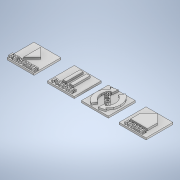
# Autodesk Inventor part: buttons
Saved by Autodesk Inventor 2022.1 (Build 261234020, 234B)
## iProperties
Created: 2021-11-01
Part Number: buttons
Material: Generico
Document SubType Name: Modeling
Designer: chicco
Density: 1 g/cm^3
Appearance: Default
Author: chicco
Autodesk Inventor part; units mm, degrees
ref_plane "YZ Plane" through (0, 0, 0) normal (1, 0, 0) x (0, 1, 0)
ref_plane "XZ Plane" through (0, 0, 0) normal (0, 1, 0) x (-1, 0, 0)
ref_plane "XY Plane" through (0, 0, 0) normal (0, 0, 1) x (1, 0, 0)
sketch "Schizzo1" plane through (0, 0, 0) normal (0, 1, 0) x (-1, 0, 0)
  line L0 (4.6852, 27.8019) -> (-9.8148, 27.8019)
  line L1 (-9.8148, 27.8019) -> (-9.8148, 13.3019)
  line L2 (-9.8148, 13.3019) -> (4.6852, 13.3019)
  line L3 (4.6852, 13.3019) -> (4.6852, 27.8019)
  line L4 (-17.0713, 27.8038) -> (-31.5713, 27.8038)
  line L5 (-31.5713, 27.8038) -> (-31.5713, 13.3038)
  line L6 (-31.5713, 13.3038) -> (-17.0713, 13.3038)
  line L7 (-17.0713, 13.3038) -> (-17.0713, 27.8038)
  line L8 (-55.7694, 27.7904) -> (-70.2694, 27.7904)
  line L9 (-70.2694, 27.7904) -> (-70.2694, 13.2904)
  line L10 (-70.2694, 13.2904) -> (-55.7694, 13.2904)
  line L11 (-55.7694, 13.2904) -> (-55.7694, 27.7904)
  line L12 (4.6852, 13.3019) -> (-76.0307, 13.3019) construction
  line L13 (-35.4166, 27.7793) -> (-49.9166, 27.7793)
  line L14 (-49.9166, 27.7793) -> (-49.9166, 13.2793)
  line L15 (-49.9166, 13.2793) -> (-35.4166, 13.2793)
  line L16 (-35.4166, 13.2793) -> (-35.4166, 27.7793)
  point P0 (0, 0)
  dimension "d0" = 14.5
  dimension "d1" = 14.5
  dimension "d6" = 14.5
  dimension "d7" = 14.5
  dimension "d8" = 14.5
  dimension "d9" = 14.5
  dimension "d10" = 14.5
  dimension "d11" = 14.5
  constraints: 34 end point, 8 parallel, 5 horizontal, 4 perpendicular
  measures "d0" distance of L2.end L1.end
  measures "d1" distance of L0.start L2.end
  measures "d6" distance of L6.end L5.end
  measures "d7" distance of L4.start L6.end
  measures "d8" distance of L10.end L9.end
  measures "d9" distance of L8.start L10.end
  measures "d10" distance of L16.start L14.end
  measures "d11" distance of L16.end L16.start
extrude "Estrusione1" add sketch "Schizzo1" along normal blind 1
sketch "Schizzo2" plane through (0, 1, 0) normal (0, 1, 0) x (1, 0, 0)
  line L0 (0.9348, -18.5902) -> (3.7499, -18.5902) construction
  line L1 (3.7499, -18.5902) -> (3.7499, -20.3496) construction
  line L2 (3.7499, -20.3496) -> (0.9348, -20.3496) construction
  line L3 (0.9348, -20.3496) -> (0.9348, -18.5902) construction
  line L4 (-7.5474, -24.5477) -> (12.5843, -24.5477) construction
  line L5 (12.5843, -24.5477) -> (12.5843, -27.7034) construction
  line L6 (12.5843, -27.7034) -> (-7.5474, -27.7034) construction
  line L7 (-7.5474, -27.7034) -> (-7.5474, -24.5477) construction
  line L8 (14.2097, -28.0868) -> (34.3415, -28.0868) construction
  line L9 (34.3415, -28.0868) -> (34.3415, -24.1124) construction
  line L10 (34.3415, -24.1124) -> (14.2097, -24.1124) construction
  line L11 (14.2097, -24.1124) -> (14.2097, -28.0868) construction
  line L12 (-3.7448, -25.0033) -> (81.6896, -25.0033) construction
  line L13 (23.1791, -18.5734) -> (25.9942, -18.5734) construction
  line L14 (25.9942, -18.5734) -> (25.9942, -20.3328) construction
  line L15 (25.9942, -20.3328) -> (23.1791, -20.3328) construction
  line L16 (23.1791, -20.3328) -> (23.1791, -18.5734) construction
  line L17 (41.3289, -21.4494) -> (41.3289, -19.69) construction
  line L18 (41.3289, -19.69) -> (44.2154, -19.69) construction
  line L19 (44.2154, -19.69) -> (44.2154, -21.4494) construction
  line L20 (44.2154, -21.4494) -> (41.3289, -21.4494) construction
  line L21 (36.8214, -12.3845) -> (34.0111, -15.1947) construction
  line L22 (34.0111, -15.1947) -> (48.2464, -29.4301) construction
  line L23 (48.2464, -29.4301) -> (51.0567, -26.6198) construction
  line L24 (51.0567, -26.6198) -> (36.8214, -12.3845) construction
  line L25 (52.8656, -24.1572) -> (52.8656, -28.1316) construction
  line L26 (52.8656, -28.1316) -> (72.9973, -28.1316) construction
  line L27 (72.9973, -28.1316) -> (72.9973, -24.1572) construction
  line L28 (72.9973, -24.1572) -> (52.8656, -24.1572) construction
  line L29 (61.9799, -18.2818) -> (61.9799, -15.4667) construction
  line L30 (61.9799, -15.4667) -> (63.7393, -15.4667) construction
  line L31 (63.7393, -15.4667) -> (63.7393, -18.2818) construction
  line L32 (63.7393, -18.2818) -> (61.9799, -18.2818) construction
  line L33 (58.2477, -18.6857) -> (58.2477, -24.1572)
  line L34 (67.3768, -24.1572) -> (67.3768, -18.6857)
  line L35 (67.3768, -18.6857) -> (58.2477, -18.6857)
  line L36 (58.2477, -24.1572) -> (67.3768, -24.1572)
  line L37 (5.1082, -19.4699) -> (0.4984, -24.0798)
  line L38 (0.4984, -24.0798) -> (0.4984, -14.8601)
  line L39 (0.4984, -14.8601) -> (5.1082, -19.4699)
  line L40 (-4.5072, -27.2255) -> (-4.5072, -25.0255)
  line L41 (-4.5072, -25.0255) -> (-3.3743, -25.0255)
  spline S0 degree 2 poles (-3.3743, -25.0255) (-3.061, -25.0255) (-2.7264, -25.1335) (-2.5231, -25.4257) (-2.5231, -25.6353) knots 0 0 0 1 2 3 3 3
  spline S1 degree 2 poles (-2.5231, -25.6353) (-2.5231, -25.8195) (-2.6798, -26.0842) (-2.8153, -26.1668) knots 0 0 0 1 2 2 2
  spline S2 degree 2 poles (-2.8153, -26.1668) (-2.9022, -26.2197) (-3.0546, -26.2536) knots 0 0 0 1 1 1
  spline S3 degree 2 poles (-3.0546, -26.2536) (-2.9339, -26.2938) (-2.8767, -26.3341) knots 0 0 0 1 1 1
  spline S4 degree 2 poles (-2.8767, -26.3341) (-2.8407, -26.3616) (-2.6989, -26.5395) (-2.6735, -26.5882) knots 0 0 0 1 2 2 2
  line L42 (-2.6735, -26.5882) -> (-2.3453, -27.2255)
  line L43 (-2.3453, -27.2255) -> (-3.1139, -27.2255)
  line L44 (-3.1139, -27.2255) -> (-3.476, -26.5522)
  spline S5 degree 2 poles (-3.476, -26.5522) (-3.5437, -26.423) (-3.5967, -26.3828) knots 0 0 0 1 1 1
  spline S6 degree 2 poles (-3.5967, -26.3828) (-3.6708, -26.332) (-3.7639, -26.332) knots 0 0 0 1 1 1
  line L45 (-3.7639, -26.332) -> (-3.8232, -26.332)
  line L46 (-3.8232, -26.332) -> (-3.8232, -27.2255)
  line L47 (-3.8232, -27.2255) -> (-4.5072, -27.2255)
  line L48 (-3.8232, -25.9169) -> (-3.5374, -25.9169)
  spline S7 degree 2 poles (-3.5374, -25.9169) (-3.4929, -25.9169) (-3.3595, -25.8873) knots 0 0 0 1 1 1
  spline S8 degree 2 poles (-3.3595, -25.8873) (-3.2918, -25.8725) (-3.2071, -25.7624) (-3.2071, -25.6904) knots 0 0 0 1 2 2 2
  spline S9 degree 2 poles (-3.2071, -25.6904) (-3.2071, -25.5845) (-3.3405, -25.4702) (-3.5268, -25.4702) knots 0 0 0 1 2 2 2
  line L49 (-3.5268, -25.4702) -> (-3.8232, -25.4702)
  line L50 (-3.8232, -25.4702) -> (-3.8232, -25.9169)
  line L51 (-2.1251, -25.0255) -> (-0.3041, -25.0255)
  line L52 (-0.3041, -25.0255) -> (-0.3041, -25.4956)
  line L53 (-0.3041, -25.4956) -> (-1.4432, -25.4956)
  line L54 (-1.4432, -25.4956) -> (-1.4432, -25.845)
  line L55 (-1.4432, -25.845) -> (-0.3867, -25.845)
  line L56 (-0.3867, -25.845) -> (-0.3867, -26.2938)
  line L57 (-0.3867, -26.2938) -> (-1.4432, -26.2938)
  line L58 (-1.4432, -26.2938) -> (-1.4432, -26.7279)
  line L59 (-1.4432, -26.7279) -> (-0.2702, -26.7279)
  line L60 (-0.2702, -26.7279) -> (-0.2702, -27.2255)
  line L61 (-0.2702, -27.2255) -> (-2.1251, -27.2255)
  line L62 (-2.1251, -27.2255) -> (-2.1251, -25.0255)
  line L63 (-0.0225, -26.4971) -> (0.6255, -26.4569)
  spline S10 degree 2 poles (0.6255, -26.4569) (0.6466, -26.6157) (0.7102, -26.6983) knots 0 0 0 1 1 1
  spline S11 degree 2 poles (0.7102, -26.6983) (0.816, -26.8317) (1.013, -26.8317) knots 0 0 0 1 1 1
  spline S12 degree 2 poles (1.013, -26.8317) (1.1569, -26.8317) (1.3158, -26.694) (1.3158, -26.6051) knots 0 0 0 1 2 2 2
  spline S13 degree 2 poles (1.3158, -26.6051) (1.3158, -26.5204) (1.2395, -26.4527) knots 0 0 0 1 1 1
  spline S14 degree 2 poles (1.2395, -26.4527) (1.1654, -26.3849) (0.8923, -26.3235) knots 0 0 0 1 1 1
  spline S15 degree 2 poles (0.8923, -26.3235) (0.4434, -26.224) (0.2528, -26.0567) knots 0 0 0 1 1 1
  spline S16 degree 2 poles (0.2528, -26.0567) (0.0601, -25.8894) (0.0601, -25.6311) knots 0 0 0 1 1 1
  spline S17 degree 2 poles (0.0601, -25.6311) (0.0601, -25.4617) (0.257, -25.161) (0.653, -24.9874) (0.996, -24.9874) knots 0 0 0 1 2 3 3 3
  spline S18 degree 2 poles (0.996, -24.9874) (1.4195, -24.9874) (1.862, -25.3008) (1.9044, -25.6438) knots 0 0 0 1 2 2 2
  line L64 (1.9044, -25.6438) -> (1.2628, -25.6819)
  spline S19 degree 2 poles (1.2628, -25.6819) (1.2374, -25.5337) (1.0722, -25.3982) (0.9283, -25.3982) knots 0 0 0 1 2 2 2
  spline S20 degree 2 poles (0.9283, -25.3982) (0.8097, -25.3982) (0.689, -25.4977) (0.689, -25.5718) knots 0 0 0 1 2 2 2
  spline S21 degree 2 poles (0.689, -25.5718) (0.689, -25.6226) (0.7398, -25.665) knots 0 0 0 1 1 1
  spline S22 degree 2 poles (0.7398, -25.665) (0.7885, -25.7094) (0.9685, -25.7454) knots 0 0 0 1 1 1
  spline S23 degree 2 poles (0.9685, -25.7454) (1.4153, -25.8428) (1.8006, -26.0398) (1.9764, -26.3298) (1.9764, -26.5098) knots 0 0 0 1 2 3 3 3
  spline S24 degree 2 poles (1.9764, -26.5098) (1.9764, -26.7216) (1.7414, -27.0794) (1.3221, -27.2636) (1.0003, -27.2636) knots 0 0 0 1 2 3 3 3
  spline S25 degree 2 poles (1.0003, -27.2636) (0.4391, -27.2636) (0.0051, -26.8317) (-0.0225, -26.4971) knots 0 0 0 1 2 2 2
  line L65 (3.7529, -25.0255) -> (4.4305, -25.0255)
  line L66 (4.4305, -25.0255) -> (4.4305, -26.3362)
  spline S26 degree 2 poles (4.4305, -26.3362) (4.4305, -26.531) (4.3098, -26.8783) (4.0493, -27.1366) (3.9054, -27.1895) knots 0 0 0 1 2 3 3 3
  spline S27 degree 2 poles (3.9054, -27.1895) (3.7084, -27.2636) (3.4289, -27.2636) knots 0 0 0 1 1 1
  spline S28 degree 2 poles (3.4289, -27.2636) (3.268, -27.2636) (2.889, -27.2192) (2.6328, -27.0858) (2.421, -26.8401) (2.3829, -26.7089) knots 0 0 0 1 2 3 4 4 4
  spline S29 degree 2 poles (2.3829, -26.7089) (2.3194, -26.4992) (2.3194, -26.3362) knots 0 0 0 1 1 1
  line L67 (2.3194, -26.3362) -> (2.3194, -25.0255)
  line L68 (2.3194, -25.0255) -> (2.997, -25.0255)
  line L69 (2.997, -25.0255) -> (2.997, -26.368)
  spline S30 degree 2 poles (2.997, -26.368) (2.997, -26.5479) (3.1981, -26.7512) (3.376, -26.7512) knots 0 0 0 1 2 2 2
  spline S31 degree 2 poles (3.376, -26.7512) (3.5517, -26.7512) (3.7529, -26.5522) (3.7529, -26.368) knots 0 0 0 1 2 2 2
  line L70 (3.7529, -26.368) -> (3.7529, -25.0255)
  line L71 (4.873, -25.0255) -> (5.7687, -25.0255)
  line L72 (5.7687, -25.0255) -> (6.1117, -26.3637)
  line L73 (6.1117, -26.3637) -> (6.4526, -25.0255)
  line L74 (6.4526, -25.0255) -> (7.3462, -25.0255)
  line L75 (7.3462, -25.0255) -> (7.3462, -27.2255)
  line L76 (7.3462, -27.2255) -> (6.7893, -27.2255)
  line L77 (6.7893, -27.2255) -> (6.7893, -25.5464)
  line L78 (6.7893, -25.5464) -> (6.3616, -27.2255)
  line L79 (6.3616, -27.2255) -> (5.8576, -27.2255)
  line L80 (5.8576, -27.2255) -> (5.4299, -25.5464)
  line L81 (5.4299, -25.5464) -> (5.4299, -27.2255)
  line L82 (5.4299, -27.2255) -> (4.873, -27.2255)
  line L83 (4.873, -27.2255) -> (4.873, -25.0255)
  line L84 (7.7824, -25.0255) -> (9.6033, -25.0255)
  line L85 (9.6033, -25.0255) -> (9.6033, -25.4956)
  line L86 (9.6033, -25.4956) -> (8.4642, -25.4956)
  line L87 (8.4642, -25.4956) -> (8.4642, -25.845)
  line L88 (8.4642, -25.845) -> (9.5208, -25.845)
  line L89 (9.5208, -25.845) -> (9.5208, -26.2938)
  line L90 (9.5208, -26.2938) -> (8.4642, -26.2938)
  line L91 (8.4642, -26.2938) -> (8.4642, -26.7279)
  line L92 (8.4642, -26.7279) -> (9.6372, -26.7279)
  line L93 (9.6372, -26.7279) -> (9.6372, -27.2255)
  line L94 (9.6372, -27.2255) -> (7.7824, -27.2255)
  line L95 (7.7824, -27.2255) -> (7.7824, -25.0255)
  line L96 (23.4846, -24.063) -> (21.6406, -24.063)
  line L97 (21.6406, -24.063) -> (21.6406, -14.8433)
  line L98 (21.6406, -14.8433) -> (23.4846, -14.8433)
  line L99 (23.4846, -14.8433) -> (23.4846, -24.063)
  line L100 (27.1724, -24.063) -> (25.3285, -24.063)
  line L101 (25.3285, -24.063) -> (25.3285, -14.8433)
  line L102 (25.3285, -14.8433) -> (27.1724, -14.8433)
  line L103 (27.1724, -14.8433) -> (27.1724, -24.063)
  line L104 (18.6888, -24.9996) -> (19.8195, -24.9996)
  spline S32 degree 2 poles (19.8195, -24.9996) (20.1879, -24.9996) (20.5563, -25.3511) (20.5563, -25.675) knots 0 0 0 1 2 2 2
  spline S33 degree 2 poles (20.5563, -25.675) (20.5563, -26.0096) (20.1561, -26.3844) (19.7454, -26.3844) knots 0 0 0 1 2 2 2
  line L105 (19.7454, -26.3844) -> (19.3727, -26.3844)
  line L106 (19.3727, -26.3844) -> (19.3727, -27.1996)
  line L107 (19.3727, -27.1996) -> (18.6888, -27.1996)
  line L108 (18.6888, -27.1996) -> (18.6888, -24.9996)
  line L109 (19.3727, -25.9376) -> (19.5379, -25.9376)
  spline S34 degree 2 poles (19.5379, -25.9376) (19.7348, -25.9376) (19.8936, -25.8) (19.8936, -25.6941) knots 0 0 0 1 2 2 2
  spline S35 degree 2 poles (19.8936, -25.6941) (19.8936, -25.5903) (19.7559, -25.4464) (19.5654, -25.4464) knots 0 0 0 1 2 2 2
  line L110 (19.5654, -25.4464) -> (19.3727, -25.4464)
  line L111 (19.3727, -25.4464) -> (19.3727, -25.9376)
  line L112 (22.2651, -26.8354) -> (21.4922, -26.8354)
  line L113 (21.4922, -26.8354) -> (21.3842, -27.1996)
  line L114 (21.3842, -27.1996) -> (20.6897, -27.1996)
  line L115 (20.6897, -27.1996) -> (21.5176, -24.9996)
  line L116 (21.5176, -24.9996) -> (22.2609, -24.9996)
  line L117 (22.2609, -24.9996) -> (23.0867, -27.1996)
  line L118 (23.0867, -27.1996) -> (22.3752, -27.1996)
  line L119 (22.3752, -27.1996) -> (22.2651, -26.8354)
  line L120 (22.1232, -26.359) -> (21.8818, -25.5692)
  line L121 (21.8818, -25.5692) -> (21.6405, -26.359)
  line L122 (21.6405, -26.359) -> (22.1232, -26.359)
  line L123 (24.7404, -24.9996) -> (25.4179, -24.9996)
  line L124 (25.4179, -24.9996) -> (25.4179, -26.3103)
  spline S36 degree 2 poles (25.4179, -26.3103) (25.4179, -26.5051) (25.2972, -26.8523) (25.0368, -27.1107) (24.8928, -27.1636) knots 0 0 0 1 2 3 3 3
  spline S37 degree 2 poles (24.8928, -27.1636) (24.6959, -27.2377) (24.4164, -27.2377) knots 0 0 0 1 1 1
  spline S38 degree 2 poles (24.4164, -27.2377) (24.2555, -27.2377) (23.8764, -27.1932) (23.6202, -27.0598) (23.4085, -26.8142) (23.3704, -26.6829) knots 0 0 0 1 2 3 4 4 4
  spline S39 degree 2 poles (23.3704, -26.6829) (23.3069, -26.4733) (23.3069, -26.3103) knots 0 0 0 1 1 1
  line L125 (23.3069, -26.3103) -> (23.3069, -24.9996)
  line L126 (23.3069, -24.9996) -> (23.9844, -24.9996)
  line L127 (23.9844, -24.9996) -> (23.9844, -26.342)
  spline S40 degree 2 poles (23.9844, -26.342) (23.9844, -26.522) (24.1856, -26.7253) (24.3635, -26.7253) knots 0 0 0 1 2 2 2
  spline S41 degree 2 poles (24.3635, -26.7253) (24.5392, -26.7253) (24.7404, -26.5262) (24.7404, -26.342) knots 0 0 0 1 2 2 2
  line L128 (24.7404, -26.342) -> (24.7404, -24.9996)
  line L129 (25.7482, -26.4712) -> (26.3962, -26.431)
  spline S42 degree 2 poles (26.3962, -26.431) (26.4174, -26.5898) (26.4809, -26.6724) knots 0 0 0 1 1 1
  spline S43 degree 2 poles (26.4809, -26.6724) (26.5867, -26.8057) (26.7837, -26.8057) knots 0 0 0 1 1 1
  spline S44 degree 2 poles (26.7837, -26.8057) (26.9277, -26.8057) (27.0865, -26.6681) (27.0865, -26.5792) knots 0 0 0 1 2 2 2
  spline S45 degree 2 poles (27.0865, -26.5792) (27.0865, -26.4945) (27.0102, -26.4267) knots 0 0 0 1 1 1
  spline S46 degree 2 poles (27.0102, -26.4267) (26.9361, -26.359) (26.663, -26.2976) knots 0 0 0 1 1 1
  spline S47 degree 2 poles (26.663, -26.2976) (26.2141, -26.198) (26.0235, -26.0308) knots 0 0 0 1 1 1
  spline S48 degree 2 poles (26.0235, -26.0308) (25.8308, -25.8635) (25.8308, -25.6052) knots 0 0 0 1 1 1
  spline S49 degree 2 poles (25.8308, -25.6052) (25.8308, -25.4358) (26.0277, -25.1351) (26.4237, -24.9615) (26.7667, -24.9615) knots 0 0 0 1 2 3 3 3
  spline S50 degree 2 poles (26.7667, -24.9615) (27.1902, -24.9615) (27.6328, -25.2749) (27.6751, -25.6179) knots 0 0 0 1 2 2 2
  line L130 (27.6751, -25.6179) -> (27.0335, -25.656)
  spline S51 degree 2 poles (27.0335, -25.656) (27.0081, -25.5078) (26.843, -25.3723) (26.699, -25.3723) knots 0 0 0 1 2 2 2
  spline S52 degree 2 poles (26.699, -25.3723) (26.5804, -25.3723) (26.4597, -25.4718) (26.4597, -25.5459) knots 0 0 0 1 2 2 2
  spline S53 degree 2 poles (26.4597, -25.5459) (26.4597, -25.5967) (26.5105, -25.6391) knots 0 0 0 1 1 1
  spline S54 degree 2 poles (26.5105, -25.6391) (26.5592, -25.6835) (26.7392, -25.7195) knots 0 0 0 1 1 1
  spline S55 degree 2 poles (26.7392, -25.7195) (27.186, -25.8169) (27.5713, -26.0138) (27.7471, -26.3039) (27.7471, -26.4839) knots 0 0 0 1 2 3 3 3
  spline S56 degree 2 poles (27.7471, -26.4839) (27.7471, -26.6956) (27.5121, -27.0535) (27.0928, -27.2377) (26.771, -27.2377) knots 0 0 0 1 2 3 3 3
  spline S57 degree 2 poles (26.771, -27.2377) (26.2098, -27.2377) (25.7758, -26.8057) (25.7482, -26.4712) knots 0 0 0 1 2 2 2
  line L131 (28.088, -24.9996) -> (29.909, -24.9996)
  line L132 (29.909, -24.9996) -> (29.909, -25.4697)
  line L133 (29.909, -25.4697) -> (28.7698, -25.4697)
  line L134 (28.7698, -25.4697) -> (28.7698, -25.819)
  line L135 (28.7698, -25.819) -> (29.8264, -25.819)
  line L136 (29.8264, -25.819) -> (29.8264, -26.2679)
  line L137 (29.8264, -26.2679) -> (28.7698, -26.2679)
  line L138 (28.7698, -26.2679) -> (28.7698, -26.702)
  line L139 (28.7698, -26.702) -> (29.9429, -26.702)
  line L140 (29.9429, -26.702) -> (29.9429, -27.1996)
  line L141 (29.9429, -27.1996) -> (28.088, -27.1996)
  line L142 (28.088, -27.1996) -> (28.088, -24.9996)
  spline S58 degree 2 poles (48.936, -20.2517) (48.936, -21.8269) (48.2903, -23.226) knots 0 0 0 1 1 1
  spline S59 degree 2 poles (48.2903, -23.226) (47.6054, -24.6838) (46.3726, -25.584) knots 0 0 0 1 1 1
  line L143 (46.3726, -25.584) -> (47.4586, -26.4352)
  line L144 (47.4586, -26.4352) -> (43.9658, -27.3744)
  line L145 (43.9658, -27.3744) -> (44.2886, -23.9011)
  line L146 (44.2886, -23.9011) -> (45.267, -24.6741)
  spline S60 degree 2 poles (45.267, -24.6741) (46.7835, -23.3337) (46.7835, -20.9464) knots 0 0 0 1 1 1
  spline S61 degree 2 poles (46.7835, -20.9464) (46.7835, -17.884) (43.8679, -16.1621) knots 0 0 0 1 1 1
  line L147 (43.8679, -16.1621) -> (45.1007, -13.765)
  spline S62 degree 2 poles (45.1007, -13.765) (46.9009, -14.6358) (47.938, -16.4556) knots 0 0 0 1 1 1
  spline S63 degree 2 poles (47.938, -16.4556) (48.936, -18.1971) (48.936, -20.2517) knots 0 0 0 1 1 1
  line L148 (41.4611, -24.9774) -> (40.2283, -27.3744)
  spline S64 degree 2 poles (40.2283, -27.3744) (38.4379, -26.5037) (37.4008, -24.6838) knots 0 0 0 1 1 1
  spline S65 degree 2 poles (37.4008, -24.6838) (36.393, -22.9423) (36.393, -20.8877) knots 0 0 0 1 1 1
  spline S66 degree 2 poles (36.393, -20.8877) (36.393, -19.3125) (37.0485, -17.9134) knots 0 0 0 1 1 1
  spline S67 degree 2 poles (37.0485, -17.9134) (37.7334, -16.4556) (38.9564, -15.5555) knots 0 0 0 1 1 1
  line L149 (38.9564, -15.5555) -> (37.8704, -14.6945)
  line L150 (37.8704, -14.6945) -> (41.3633, -13.765)
  line L151 (41.3633, -13.765) -> (41.0404, -17.2383)
  line L152 (41.0404, -17.2383) -> (40.062, -16.4654)
  spline S68 degree 2 poles (40.062, -16.4654) (38.5455, -17.8058) (38.5455, -20.193) knots 0 0 0 1 1 1
  spline S69 degree 2 poles (38.5455, -20.193) (38.5455, -23.2554) (41.4611, -24.9774) knots 0 0 0 1 1 1
  line L153 (39.0842, -17.9831) -> (39.5708, -18.4128)
  spline S70 degree 2 poles (39.5708, -18.4128) (39.4735, -18.5401) (39.46, -18.6434) knots 0 0 0 1 1 1
  spline S71 degree 2 poles (39.46, -18.6434) (39.4406, -18.8126) (39.5798, -18.9519) knots 0 0 0 1 1 1
  spline S72 degree 2 poles (39.5798, -18.9519) (39.6816, -19.0537) (39.8912, -19.0686) (39.9541, -19.0058) knots 0 0 0 1 2 2 2
  spline S73 degree 2 poles (39.9541, -19.0058) (40.014, -18.9459) (40.008, -18.8441) knots 0 0 0 1 1 1
  spline S74 degree 2 poles (40.008, -18.8441) (40.0035, -18.7437) (39.8538, -18.5072) knots 0 0 0 1 1 1
  spline S75 degree 2 poles (39.8538, -18.5072) (39.6068, -18.1194) (39.5903, -17.8664) knots 0 0 0 1 1 1
  spline S76 degree 2 poles (39.5903, -17.8664) (39.5723, -17.6118) (39.755, -17.4292) knots 0 0 0 1 1 1
  spline S77 degree 2 poles (39.755, -17.4292) (39.8748, -17.3094) (40.2266, -17.236) (40.6294, -17.3932) (40.8719, -17.6358) knots 0 0 0 1 2 3 3 3
  spline S78 degree 2 poles (40.8719, -17.6358) (41.1714, -17.9352) (41.2627, -18.4697) (41.0501, -18.7422) knots 0 0 0 1 2 2 2
  line L154 (41.0501, -18.7422) -> (40.5695, -18.3155)
  spline S79 degree 2 poles (40.5695, -18.3155) (40.6563, -18.1928) (40.6354, -17.9801) (40.5336, -17.8783) knots 0 0 0 1 2 2 2
  spline S80 degree 2 poles (40.5336, -17.8783) (40.4497, -17.7945) (40.294, -17.7795) (40.2416, -17.8319) knots 0 0 0 1 2 2 2
  spline S81 degree 2 poles (40.2416, -17.8319) (40.2057, -17.8678) (40.2117, -17.9337) knots 0 0 0 1 1 1
  spline S82 degree 2 poles (40.2117, -17.9337) (40.2146, -17.9996) (40.3165, -18.1523) knots 0 0 0 1 1 1
  spline S83 degree 2 poles (40.3165, -18.1523) (40.5635, -18.5371) (40.6968, -18.9489) (40.6159, -19.2783) (40.4886, -19.4055) knots 0 0 0 1 2 3 3 3
  spline S84 degree 2 poles (40.4886, -19.4055) (40.3389, -19.5552) (39.9197, -19.6421) (39.493, -19.4759) (39.2654, -19.2483) knots 0 0 0 1 2 3 3 3
  spline S85 degree 2 poles (39.2654, -19.2483) (38.8686, -18.8515) (38.8671, -18.2392) (39.0842, -17.9831) knots 0 0 0 1 2 2 2
  line L155 (41.67, -18.4877) -> (43.1328, -19.9505)
  line L156 (43.1328, -19.9505) -> (42.748, -20.3353)
  line L157 (42.748, -20.3353) -> (42.2569, -19.8442)
  line L158 (42.2569, -19.8442) -> (41.086, -21.0151)
  line L159 (41.086, -21.0151) -> (40.6054, -20.5344)
  line L160 (40.6054, -20.5344) -> (41.7763, -19.3636)
  line L161 (41.7763, -19.3636) -> (41.2852, -18.8725)
  line L162 (41.2852, -18.8725) -> (41.67, -18.4877)
  spline S86 degree 2 poles (42.5114, -20.8863) (42.8917, -20.506) (43.7421, -20.506) (44.121, -20.8848) knots 0 0 0 1 2 2 2
  spline S87 degree 2 poles (44.121, -20.8848) (44.5087, -21.2726) (44.5117, -22.111) (44.1359, -22.4868) knots 0 0 0 1 2 2 2
  spline S88 degree 2 poles (44.1359, -22.4868) (43.8634, -22.7593) (43.3304, -22.924) (42.7884, -22.7713) (42.5294, -22.5123) knots 0 0 0 1 2 3 3 3
  spline S89 degree 2 poles (42.5294, -22.5123) (42.2674, -22.2503) (42.0892, -21.7367) (42.2389, -21.1588) (42.5114, -20.8863) knots 0 0 0 1 2 3 3 3
  spline S90 degree 2 poles (42.989, -21.3699) (42.754, -21.605) (42.7225, -21.9868) (42.8737, -22.138) knots 0 0 0 1 2 2 2
  spline S91 degree 2 poles (42.8737, -22.138) (43.028, -22.2922) (43.4008, -22.2608) (43.6613, -22.0002) knots 0 0 0 1 2 2 2
  spline S92 degree 2 poles (43.6613, -22.0002) (43.8814, -21.7801) (43.9083, -21.3998) (43.7556, -21.2471) knots 0 0 0 1 2 2 2
  spline S93 degree 2 poles (43.7556, -21.2471) (43.6104, -21.1019) (43.2271, -21.1318) (42.989, -21.3699) knots 0 0 0 1 2 2 2
  line L163 (45.16, -21.9778) -> (45.9596, -22.7773)
  spline S94 degree 2 poles (45.9596, -22.7773) (46.2201, -23.0378) (46.2321, -23.5469) (46.003, -23.776) knots 0 0 0 1 2 2 2
  spline S95 degree 2 poles (46.003, -23.776) (45.7664, -24.0125) (45.2184, -23.9946) (44.928, -23.7041) knots 0 0 0 1 2 2 2
  line L164 (44.928, -23.7041) -> (44.6644, -23.4406)
  line L165 (44.6644, -23.4406) -> (44.088, -24.017)
  line L166 (44.088, -24.017) -> (43.6044, -23.5334)
  line L167 (43.6044, -23.5334) -> (45.16, -21.9778)
  line L168 (44.9804, -23.1247) -> (45.0972, -23.2415)
  spline S96 degree 2 poles (45.0972, -23.2415) (45.2364, -23.3807) (45.446, -23.3957) (45.5209, -23.3208) knots 0 0 0 1 2 2 2
  spline S97 degree 2 poles (45.5209, -23.3208) (45.5942, -23.2474) (45.5987, -23.0483) (45.464, -22.9136) knots 0 0 0 1 2 2 2
  line L169 (45.464, -22.9136) -> (45.3277, -22.7773)
  line L170 (45.3277, -22.7773) -> (44.9804, -23.1247)
  line L171 (62.8596, -14.1084) -> (67.4694, -18.7182)
  line L172 (67.4694, -18.7182) -> (58.2497, -18.7182)
  line L173 (58.2497, -18.7182) -> (62.8596, -14.1084)
  line L174 (58.036, -25.0444) -> (58.7157, -25.0444)
  line L175 (58.7157, -25.0444) -> (58.7157, -25.8152)
  line L176 (58.7157, -25.8152) -> (59.4589, -25.8152)
  line L177 (59.4589, -25.8152) -> (59.4589, -25.0444)
  line L178 (59.4589, -25.0444) -> (60.1428, -25.0444)
  line L179 (60.1428, -25.0444) -> (60.1428, -27.2444)
  line L180 (60.1428, -27.2444) -> (59.4589, -27.2444)
  line L181 (59.4589, -27.2444) -> (59.4589, -26.3551)
  line L182 (59.4589, -26.3551) -> (58.7157, -26.3551)
  line L183 (58.7157, -26.3551) -> (58.7157, -27.2444)
  line L184 (58.7157, -27.2444) -> (58.036, -27.2444)
  line L185 (58.036, -27.2444) -> (58.036, -25.0444)
  spline S98 degree 2 poles (60.5091, -26.1455) (60.5091, -25.6077) (61.1105, -25.0063) (61.6462, -25.0063) knots 0 0 0 1 2 2 2
  spline S99 degree 2 poles (61.6462, -25.0063) (62.1946, -25.0063) (62.7896, -25.5971) (62.7896, -26.1285) knots 0 0 0 1 2 2 2
  spline S100 degree 2 poles (62.7896, -26.1285) (62.7896, -26.5139) (62.5291, -27.0073) (62.0379, -27.2825) (61.6716, -27.2825) knots 0 0 0 1 2 3 3 3
  spline S101 degree 2 poles (61.6716, -27.2825) (61.301, -27.2825) (60.8119, -27.0454) (60.5091, -26.5309) (60.5091, -26.1455) knots 0 0 0 1 2 3 3 3
  spline S102 degree 2 poles (61.1888, -26.1497) (61.1888, -26.4822) (61.4365, -26.7744) (61.6504, -26.7744) knots 0 0 0 1 2 2 2
  spline S103 degree 2 poles (61.6504, -26.7744) (61.8685, -26.7744) (62.1099, -26.4885) (62.1099, -26.1201) knots 0 0 0 1 2 2 2
  spline S104 degree 2 poles (62.1099, -26.1201) (62.1099, -25.8088) (61.86, -25.5208) (61.644, -25.5208) knots 0 0 0 1 2 2 2
  spline S105 degree 2 poles (61.644, -25.5208) (61.4387, -25.5208) (61.1888, -25.813) (61.1888, -26.1497) knots 0 0 0 1 2 2 2
  line L186 (63.1495, -25.0444) -> (64.0452, -25.0444)
  line L187 (64.0452, -25.0444) -> (64.3882, -26.3826)
  line L188 (64.3882, -26.3826) -> (64.7291, -25.0444)
  line L189 (64.7291, -25.0444) -> (65.6227, -25.0444)
  line L190 (65.6227, -25.0444) -> (65.6227, -27.2444)
  line L191 (65.6227, -27.2444) -> (65.0658, -27.2444)
  line L192 (65.0658, -27.2444) -> (65.0658, -25.5653)
  line L193 (65.0658, -25.5653) -> (64.6381, -27.2444)
  line L194 (64.6381, -27.2444) -> (64.1341, -27.2444)
  line L195 (64.1341, -27.2444) -> (63.7064, -25.5653)
  line L196 (63.7064, -25.5653) -> (63.7064, -27.2444)
  line L197 (63.7064, -27.2444) -> (63.1495, -27.2444)
  line L198 (63.1495, -27.2444) -> (63.1495, -25.0444)
  line L199 (66.0589, -25.0444) -> (67.8798, -25.0444)
  line L200 (67.8798, -25.0444) -> (67.8798, -25.5145)
  line L201 (67.8798, -25.5145) -> (66.7407, -25.5145)
  line L202 (66.7407, -25.5145) -> (66.7407, -25.8639)
  line L203 (66.7407, -25.8639) -> (67.7973, -25.8639)
  line L204 (67.7973, -25.8639) -> (67.7973, -26.3128)
  line L205 (67.7973, -26.3128) -> (66.7407, -26.3128)
  line L206 (66.7407, -26.3128) -> (66.7407, -26.7468)
  line L207 (66.7407, -26.7468) -> (67.9137, -26.7468)
  line L208 (67.9137, -26.7468) -> (67.9137, -27.2444)
  line L209 (67.9137, -27.2444) -> (66.0589, -27.2444)
  line L210 (66.0589, -27.2444) -> (66.0589, -25.0444)
  point P0 (0, 0)
  constraints: 10 end point, 2 point on line, 2 vertical, 1 collinear, 1 horizontal, 1 perpendicular, 16 other
extrude "Estrusione2" add sketch "Schizzo2" along normal blind 1
